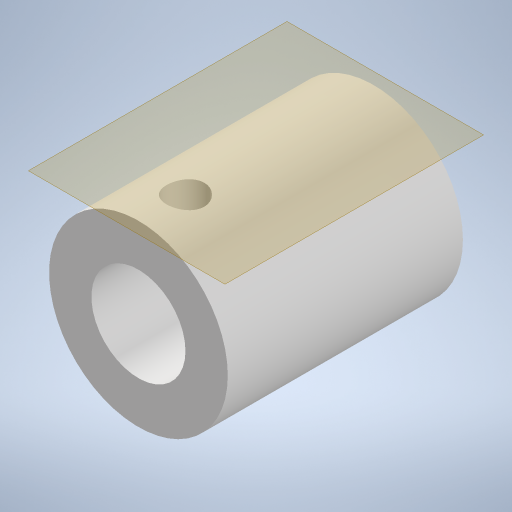
# Autodesk Inventor part: handleAdapter
Saved by Autodesk Inventor 2024.2 (Build 282272000, 272)
## iProperties
Created: 2024-06-01
Part Number: handleAdapter
Material: Generic
Document SubType Name: Modeling
Designer: user
Density: 1 g/cm^3
Appearance: Default
Author: user
Autodesk Inventor part; units mm, degrees
ref_plane "YZ Plane" through (0, 0, 0) normal (1, 0, 0) x (0, 1, 0)
ref_plane "XY Plane" through (0, 0, 0) normal (0, 0, 1) x (1, 0, 0)
sketch "Sketch1" plane through (0, 0, 0) normal (0, 0, 1) x (1, 0, 0)
  circle A0 centre (0, 0) radius 9.5
  dimension "d0" = 19
  constraints: 1 centre point, 1 coincident
  measures "d0" diameter of A0
extrude "Extrusion1" add sketch "Sketch1" along normal blind 25
sketch "Sketch2" plane through (0, 0, 25) normal (0, 0, 1) x (1, 0, 0)
  point P0 (0, 0)
  point P1 (0, 0)
  constraints: 1 coincident
hole "Hole1" at (0, 0, 25) direction (0, 0, -1) diameter 10 depth 8 tip angle 118
sketch "Sketch3" plane through (0, 0, 0) normal (0, 0, -1) x (-1, 0, 0)
  point P0 (0, 0)
  point P1 (0, 0)
  constraints: 1 coincident
hole "Hole2" at (0, 0, 0) direction (0, 0, 1) diameter 12 depth 8 tip angle 118
sketch "Sketch4" plane through (0, 0, 0) normal (0, 1, 0) x (-1, 0, 0)
  line L0 (9.5, 25) -> (-9.5, 25) projected
  circle A0 centre (0, 20) radius 2
  point P0 (0, 0)
  dimension "d17" = 5
  dimension "d18" = 4
  constraints: 1 centre point, 1 coincident
  measures "d17" distance from line of L0 point (0, 20)
  measures "d18" diameter of A0
extrude "Extrusion2" cut sketch "Sketch4" along normal through all
ref_plane "Work Plane1" through (0, 9.5, 0) normal (0, 1, 0) x (-1, 0, 0)
body "Solid1"
